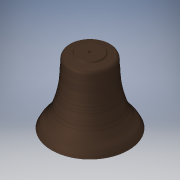
# Autodesk Inventor part: bell
Saved by Autodesk Inventor 2017 (Build 210142000, 142)
## iProperties
Created: 2016-09-29
Part Number: bell
Material: Bronze, Cast
Document SubType Name: Modeling
Designer: canti021
Density: 8.45 g/cm^3
Appearance: Bronze - Satin
Author: canti021
Autodesk Inventor part; units mm, degrees
ref_plane "YZ Plane" through (0, 0, 0) normal (1, 0, 0) x (0, 1, 0)
ref_plane "XZ Plane" through (0, 0, 0) normal (0, 1, 0) x (-1, 0, 0)
ref_plane "XY Plane" through (0, 0, 0) normal (0, 0, 1) x (1, 0, 0)
sketch "Sketch1" plane through (0, 0, 0) normal (0, 0, 1) x (1, 0, 0)
  spline S0 degree 3 poles (58.871, 16.2187) (58.8456, 16.6364) (59.2227, 17.7302) (62.2401, 23.533) (64.3081, 27.5098) (66, 31.0198) (66, 31.3331) (66, 31.6465) (68.4469, 36.5488) (71.4375, 42.2273) (76.7576, 52.3288) (77.7094, 54.0452) (83.4201, 63.8339) (84.9574, 66.469) (90.7691, 73.7771) (96.3349, 80.0741) (106.446, 91.5134) (114.75, 101.5516) (114.75, 102.335) (114.75, 102.5632) (115.2804, 103.3406) (115.9287, 104.0625) (117.7509, 106.0915) (128.1618, 122.2601) (129.8128, 125.625) (130.6224, 127.275) (132.2051, 130.0773) (133.3299, 131.8523) (137.2192, 137.9897) (150.75, 163.3632) (150.75, 164.5191) (150.75, 164.8886) (151.7405, 167.2573) (152.951, 169.783) (155.5846, 175.2773) (161.25, 190.7483) (161.25, 192.4455) (161.25, 193.1071) (161.7267, 194.7118) (162.3093, 196.0117) (162.8919, 197.3115) (164.1292, 201.4125) (165.0589, 205.125) (165.9886, 208.8375) (167.0014, 212.2125) (167.3095, 212.625) (167.6177, 213.0375) (168.591, 216.3598) (169.4725, 220.0078) (170.3539, 223.6558) (171.359, 227.1996) (171.706, 227.8828) (172.555, 229.5544) (174.7488, 237.242) (174.7546, 238.5659) (174.757, 239.1484) (175.2636, 240.592) (175.88, 241.7739) (176.4963, 242.9557) (177.6864, 246.837) (178.5246, 250.3989) (179.3627, 253.9607) (180.3404, 257.55) (180.6973, 258.375) (181.3815, 259.9569) (182.4138, 264.9065) (183.7475, 273) (184.1893, 275.6812) (184.8551, 278.55) (185.2271, 279.375) (185.599, 280.2) (186.6498, 285.0938) (187.5622, 290.25) (188.4745, 295.4062) (189.4794, 299.9625) (189.7952, 300.375) (190.111, 300.7875) (191.11, 306.3562) (192.0153, 312.75) (192.9205, 319.1438) (193.9326, 324.7125) (194.2645, 325.125) (194.5964, 325.5375) (195.244, 328.575) (195.7037, 331.875) (196.9806, 341.041) (198.6765, 352.8509) (199.8503, 360.75) (200.4326, 364.6688) (201.3057, 374.625) (201.7907, 382.875) (202.2756, 391.125) (202.9691, 398.4399) (203.3319, 399.1302) (203.6947, 399.8206) (204.6695, 416.9551) (205.4982, 437.2069) (206.327, 457.4587) (207.3134, 474.6126) (207.6904, 475.3267) (208.0675, 476.0408) (208.7597, 486.4125) (209.2287, 498.375) (210.504, 530.9028) (211.2343, 542.5727) (212.0952, 544.1776) (212.5221, 544.9737) (213.6114, 547.4813) (214.5157, 549.75) (216.8217, 555.5352) (221.1847, 561.067) (225.8758, 564.1535) (229.4678, 566.5169) (230.7149, 566.876) (238.125, 567.6802) (242.6625, 568.1727) (247.3875, 568.8781) (248.625, 569.2477) (249.8625, 569.6174) (257.2875, 570.6295) (265.125, 571.4968) (282.6702, 573.4384) (285.3766, 574.4859) (287.4793, 580.1489) (288.2336, 582.1805) (289.2088, 584.2742) (289.6466, 584.8016) (290.2812, 585.5662) (300.6399, 585.7215) (340.7837, 585.5677) (357.5641, 585.5035) (374.3446, 585.4392) (391.125, 585.375) (391.125, 581.7967) (391.125, 578.2456) (391.125, 574.6824) (391.125, 571.1192) (391.125, 567.5645) (391.125, 563.9878) (376.9718, 563.9894) (362.4025, 563.9788) (347.8331, 563.9682) (333.2637, 563.9576) (318.6944, 563.947) (304.125, 563.9364) (303.375, 562.426) (302.625, 560.9155) (301.875, 559.405) (300.6375, 556.9128) (299.2875, 554.5967) (298.875, 554.2583) (297.0424, 552.7548) (281.0236, 551.2893) (261, 550.7932) (253.875, 550.6167) (246.75, 550.4402) (239.625, 550.2637) (238.4663, 549.2882) (237.3075, 548.3127) (236.1488, 547.3372) (233.3231, 544.9584) (232.446, 543.6029) (231.4613, 540.0937) (230.7951, 537.7193) (230.25, 534.6797) (230.25, 533.339) (230.25, 531.9983) (229.9145, 530.2745) (229.5045, 529.5084) (229.0945, 528.7422) (228.21, 515.6863) (227.539, 500.4952) (226.868, 485.3041) (226.0173, 467.9812) (225.6487, 462) (225.28, 456.0188) (224.6956, 446.5688) (224.35, 441) (224.0044, 435.4312) (223.1662, 417.5438) (222.4875, 401.25) (221.8087, 384.9562) (220.9394, 370.4438) (220.5558, 369) (220.1721, 367.5562) (219.4736, 360.975) (219.0035, 354.375) (217.773, 337.0987) (216.3606, 322.3014) (215.8179, 321) (215.5598, 320.3812) (214.6315, 313.4625) (213.7549, 305.625) (212.8783, 297.7875) (211.8736, 290.7) (211.5221, 289.875) (210.8262, 288.2412) (209.4857, 280.6339) (208.1954, 270.9971) (207.7442, 267.6268) (207.1219, 264.6174) (206.8125, 264.3096) (206.5031, 264.0018) (206.25, 262.9976) (206.25, 262.078) (206.25, 259.787) (203.3245, 244.4781) (202.5325, 242.625) (201.713, 240.7073) (198.4367, 227.761) (196.0792, 217.125) (195.0735, 212.5875) (193.9209, 208.2) (193.5177, 207.375) (193.1146, 206.55) (192.0614, 203.021) (191.1772, 199.5329) (190.293, 196.0447) (189.3074, 192.6697) (188.9869, 192.0329) (188.6665, 191.396) (187.5573, 187.1625) (186.5221, 182.625) (184.5781, 174.1044) (181.7392, 163.8658) (177.8918, 151.5) (176.6726, 147.5812) (174.7608, 141.3375) (173.6434, 137.625) (172.526, 133.9125) (171.3569, 130.5375) (171.0454, 130.125) (170.7338, 129.7125) (169.8961, 127.5188) (169.1837, 125.25) (167.9712, 121.3882) (160.907, 104.0319) (157.126, 95.625) (156.1984, 93.5625) (155.0081, 90.525) (154.481, 88.875) (153.9538, 87.225) (153.1026, 85.2) (152.5894, 84.375) (152.0761, 83.55) (151.4054, 82.0312) (151.0988, 81) (150.7922, 79.9688) (148.9852, 76.3085) (147.0832, 72.8661) (145.1812, 69.4237) (141.6, 62.7675) (139.125, 58.0745) (136.65, 53.3815) (132.2821, 46.1097) (129.4185, 41.915) (124.941, 35.3561) (123.7334, 34.0892) (120.7935, 32.8663) (118.9133, 32.0843) (116.3625, 30.9613) (115.125, 30.3708) (113.8875, 29.7804) (110.85, 28.5885) (108.375, 27.7223) (105.9, 26.8562) (102.6348, 25.4882) (101.119, 24.6825) (97.8316, 22.9351) (89.7823, 20.718) (78, 18.3146) (68.7056, 16.4187) (64.2733, 15.411) (61.8226, 14.6364) (60.8676, 14.3345) (59.9258, 14.5607) (59.3753, 15.2241) (59.3753, 15.2241) (58.8964, 15.801) (58.871, 16.2187) knots 3 3 3 3 4 5 6 7 8 9 10 11 12 13 14 15 16 17 18 19 20 21 22 23 24 25 26 27 28 29 30 31 32 33 34 35 36 37 38 39 40 41 42 43 44 45 46 47 48 49 50 51 52 53 54 55 56 57 58 59 60 61 62 63 64 65 66 67 68 69 70 71 72 73 74 75 76 77 78 79 80 81 82 83 84 85 86 87 88 89 90 91 92 93 94 95 96 97 98 99 100 101 102 103 104 105 106 107 108 109 110 111 112 113 114 115 116 117 118 119 120 121 122 123 124 125 126 127 128 129 130 131 132 133 134 135 136 137 138 139 140 141 142 143 144 145 146 147 148 149 150 151 152 153 154 155 156 157 158 159 160 161 162 163 164 165 166 167 168 169 170 171 172 173 174 175 176 177 178 179 180 181 182 183 184 185 186 187 188 189 190 191 192 193 194 195 196 197 198 199 200 201 202 203 204 205 206 207 208 209 210 211 212 213 214 215 216 217 218 219 220 221 222 223 224 225 226 227 228 229 230 231 232 233 234 235 236 237 238 239 240 241 242 243 244 245 246 247 248 249 250 251 252 253 254 255 256 257 258 259 260 261 262 263 264 265 266 267 268 269 270 271 272 273 274 275 276 277 278 279 280 280 280 280
  line L0 (58.871, 16.2187) -> (58.8456, 16.6364) construction
  line L1 (58.8456, 16.6364) -> (59.2227, 17.7302) construction
  line L2 (59.2227, 17.7302) -> (62.2401, 23.533) construction
  line L3 (62.2401, 23.533) -> (64.3081, 27.5098) construction
  line L4 (64.3081, 27.5098) -> (66, 31.0198) construction
  line L5 (66, 31.0198) -> (66, 31.3331) construction
  line L6 (66, 31.3331) -> (66, 31.6465) construction
  line L7 (66, 31.6465) -> (68.4469, 36.5488) construction
  line L8 (68.4469, 36.5488) -> (71.4375, 42.2273) construction
  line L9 (71.4375, 42.2273) -> (76.7576, 52.3288) construction
  line L10 (76.7576, 52.3288) -> (77.7094, 54.0452) construction
  line L11 (77.7094, 54.0452) -> (83.4201, 63.8339) construction
  line L12 (83.4201, 63.8339) -> (84.9574, 66.469) construction
  line L13 (84.9574, 66.469) -> (90.7691, 73.7771) construction
  line L14 (90.7691, 73.7771) -> (96.3349, 80.0741) construction
  line L15 (96.3349, 80.0741) -> (106.446, 91.5134) construction
  line L16 (106.446, 91.5134) -> (114.75, 101.5516) construction
  line L17 (114.75, 101.5516) -> (114.75, 102.335) construction
  line L18 (114.75, 102.335) -> (114.75, 102.5632) construction
  line L19 (114.75, 102.5632) -> (115.2804, 103.3406) construction
  line L20 (115.2804, 103.3406) -> (115.9287, 104.0625) construction
  line L21 (115.9287, 104.0625) -> (117.7509, 106.0915) construction
  line L22 (117.7509, 106.0915) -> (128.1618, 122.2601) construction
  line L23 (128.1618, 122.2601) -> (129.8128, 125.625) construction
  line L24 (129.8128, 125.625) -> (130.6224, 127.275) construction
  line L25 (130.6224, 127.275) -> (132.2051, 130.0773) construction
  line L26 (132.2051, 130.0773) -> (133.3299, 131.8523) construction
  line L27 (133.3299, 131.8523) -> (137.2192, 137.9897) construction
  line L28 (137.2192, 137.9897) -> (150.75, 163.3632) construction
  line L29 (150.75, 163.3632) -> (150.75, 164.5191) construction
  line L30 (150.75, 164.5191) -> (150.75, 164.8886) construction
  line L31 (150.75, 164.8886) -> (151.7405, 167.2573) construction
  line L32 (151.7405, 167.2573) -> (152.951, 169.783) construction
  line L33 (152.951, 169.783) -> (155.5846, 175.2773) construction
  line L34 (155.5846, 175.2773) -> (161.25, 190.7483) construction
  line L35 (161.25, 190.7483) -> (161.25, 192.4455) construction
  line L36 (161.25, 192.4455) -> (161.25, 193.1071) construction
  line L37 (161.25, 193.1071) -> (161.7267, 194.7118) construction
  line L38 (161.7267, 194.7118) -> (162.3093, 196.0117) construction
  line L39 (162.3093, 196.0117) -> (162.8919, 197.3115) construction
  line L40 (162.8919, 197.3115) -> (164.1292, 201.4125) construction
  line L41 (164.1292, 201.4125) -> (165.0589, 205.125) construction
  line L42 (165.0589, 205.125) -> (165.9886, 208.8375) construction
  line L43 (165.9886, 208.8375) -> (167.0014, 212.2125) construction
  line L44 (167.0014, 212.2125) -> (167.3095, 212.625) construction
  line L45 (167.3095, 212.625) -> (167.6177, 213.0375) construction
  line L46 (167.6177, 213.0375) -> (168.591, 216.3598) construction
  line L47 (168.591, 216.3598) -> (169.4725, 220.0078) construction
  line L48 (169.4725, 220.0078) -> (170.3539, 223.6558) construction
  line L49 (170.3539, 223.6558) -> (171.359, 227.1996) construction
  line L50 (171.359, 227.1996) -> (171.706, 227.8828) construction
  line L51 (171.706, 227.8828) -> (172.555, 229.5544) construction
  line L52 (172.555, 229.5544) -> (174.7488, 237.242) construction
  line L53 (174.7488, 237.242) -> (174.7546, 238.5659) construction
  line L54 (174.7546, 238.5659) -> (174.757, 239.1484) construction
  line L55 (174.757, 239.1484) -> (175.2636, 240.592) construction
  line L56 (175.2636, 240.592) -> (175.88, 241.7739) construction
  line L57 (175.88, 241.7739) -> (176.4963, 242.9557) construction
  line L58 (176.4963, 242.9557) -> (177.6864, 246.837) construction
  line L59 (177.6864, 246.837) -> (178.5246, 250.3989) construction
  line L60 (178.5246, 250.3989) -> (179.3627, 253.9607) construction
  line L61 (179.3627, 253.9607) -> (180.3404, 257.55) construction
  line L62 (180.3404, 257.55) -> (180.6973, 258.375) construction
  line L63 (180.6973, 258.375) -> (181.3815, 259.9569) construction
  line L64 (181.3815, 259.9569) -> (182.4138, 264.9065) construction
  line L65 (182.4138, 264.9065) -> (183.7475, 273) construction
  line L66 (183.7475, 273) -> (184.1893, 275.6812) construction
  line L67 (184.1893, 275.6812) -> (184.8551, 278.55) construction
  line L68 (184.8551, 278.55) -> (185.2271, 279.375) construction
  line L69 (185.2271, 279.375) -> (185.599, 280.2) construction
  line L70 (185.599, 280.2) -> (186.6498, 285.0938) construction
  line L71 (186.6498, 285.0938) -> (187.5622, 290.25) construction
  line L72 (187.5622, 290.25) -> (188.4745, 295.4062) construction
  line L73 (188.4745, 295.4062) -> (189.4794, 299.9625) construction
  line L74 (189.4794, 299.9625) -> (189.7952, 300.375) construction
  line L75 (189.7952, 300.375) -> (190.111, 300.7875) construction
  line L76 (190.111, 300.7875) -> (191.11, 306.3562) construction
  line L77 (191.11, 306.3562) -> (192.0153, 312.75) construction
  line L78 (192.0153, 312.75) -> (192.9205, 319.1438) construction
  line L79 (192.9205, 319.1438) -> (193.9326, 324.7125) construction
  line L80 (193.9326, 324.7125) -> (194.2645, 325.125) construction
  line L81 (194.2645, 325.125) -> (194.5964, 325.5375) construction
  line L82 (194.5964, 325.5375) -> (195.244, 328.575) construction
  line L83 (195.244, 328.575) -> (195.7037, 331.875) construction
  line L84 (195.7037, 331.875) -> (196.9806, 341.041) construction
  line L85 (196.9806, 341.041) -> (198.6765, 352.8509) construction
  line L86 (198.6765, 352.8509) -> (199.8503, 360.75) construction
  line L87 (199.8503, 360.75) -> (200.4326, 364.6688) construction
  line L88 (200.4326, 364.6688) -> (201.3057, 374.625) construction
  line L89 (201.3057, 374.625) -> (201.7907, 382.875) construction
  line L90 (201.7907, 382.875) -> (202.2756, 391.125) construction
  line L91 (202.2756, 391.125) -> (202.9691, 398.4399) construction
  line L92 (202.9691, 398.4399) -> (203.3319, 399.1302) construction
  line L93 (203.3319, 399.1302) -> (203.6947, 399.8206) construction
  line L94 (203.6947, 399.8206) -> (204.6695, 416.9551) construction
  line L95 (204.6695, 416.9551) -> (205.4982, 437.2069) construction
  line L96 (205.4982, 437.2069) -> (206.327, 457.4587) construction
  line L97 (206.327, 457.4587) -> (207.3134, 474.6126) construction
  line L98 (207.3134, 474.6126) -> (207.6904, 475.3267) construction
  line L99 (207.6904, 475.3267) -> (208.0675, 476.0408) construction
  line L100 (208.0675, 476.0408) -> (208.7597, 486.4125) construction
  line L101 (208.7597, 486.4125) -> (209.2287, 498.375) construction
  line L102 (209.2287, 498.375) -> (210.504, 530.9028) construction
  line L103 (210.504, 530.9028) -> (211.2343, 542.5727) construction
  line L104 (211.2343, 542.5727) -> (212.0952, 544.1776) construction
  line L105 (212.0952, 544.1776) -> (212.5221, 544.9737) construction
  line L106 (212.5221, 544.9737) -> (213.6114, 547.4813) construction
  line L107 (213.6114, 547.4813) -> (214.5157, 549.75) construction
  line L108 (214.5157, 549.75) -> (216.8217, 555.5352) construction
  line L109 (216.8217, 555.5352) -> (221.1847, 561.067) construction
  line L110 (221.1847, 561.067) -> (225.8758, 564.1535) construction
  line L111 (225.8758, 564.1535) -> (229.4678, 566.5169) construction
  line L112 (229.4678, 566.5169) -> (230.7149, 566.876) construction
  line L113 (230.7149, 566.876) -> (238.125, 567.6802) construction
  line L114 (238.125, 567.6802) -> (242.6625, 568.1727) construction
  line L115 (242.6625, 568.1727) -> (247.3875, 568.8781) construction
  line L116 (247.3875, 568.8781) -> (248.625, 569.2477) construction
  line L117 (248.625, 569.2477) -> (249.8625, 569.6174) construction
  line L118 (249.8625, 569.6174) -> (257.2875, 570.6295) construction
  line L119 (257.2875, 570.6295) -> (265.125, 571.4968) construction
  line L120 (265.125, 571.4968) -> (282.6702, 573.4384) construction
  line L121 (282.6702, 573.4384) -> (285.3766, 574.4859) construction
  line L122 (285.3766, 574.4859) -> (287.4793, 580.1489) construction
  line L123 (287.4793, 580.1489) -> (288.2336, 582.1805) construction
  line L124 (288.2336, 582.1805) -> (289.2088, 584.2742) construction
  line L125 (289.2088, 584.2742) -> (289.6466, 584.8016) construction
  line L126 (289.6466, 584.8016) -> (290.2812, 585.5662) construction
  line L127 (290.2812, 585.5662) -> (300.6399, 585.7215) construction
  line L128 (300.6399, 585.7215) -> (340.7837, 585.5677) construction
  line L129 (340.7837, 585.5677) -> (357.5641, 585.5035) construction
  line L130 (357.5641, 585.5035) -> (374.3446, 585.4392) construction
  line L131 (374.3446, 585.4392) -> (391.125, 585.375) construction
  line L132 (391.125, 585.375) -> (391.125, 581.7967) construction
  line L133 (391.125, 581.7967) -> (391.125, 578.2456) construction
  line L134 (391.125, 578.2456) -> (391.125, 574.6824) construction
  line L135 (391.125, 574.6824) -> (391.125, 571.1192) construction
  line L136 (391.125, 571.1192) -> (391.125, 567.5645) construction
  line L137 (391.125, 567.5645) -> (391.125, 563.9878) construction
  line L138 (391.125, 563.9878) -> (376.9718, 563.9894) construction
  line L139 (376.9718, 563.9894) -> (362.4025, 563.9788) construction
  line L140 (362.4025, 563.9788) -> (347.8331, 563.9682) construction
  line L141 (347.8331, 563.9682) -> (333.2637, 563.9576) construction
  line L142 (333.2637, 563.9576) -> (318.6944, 563.947) construction
  line L143 (318.6944, 563.947) -> (304.125, 563.9364) construction
  line L144 (304.125, 563.9364) -> (303.375, 562.426) construction
  line L145 (303.375, 562.426) -> (302.625, 560.9155) construction
  line L146 (302.625, 560.9155) -> (301.875, 559.405) construction
  line L147 (301.875, 559.405) -> (300.6375, 556.9128) construction
  line L148 (300.6375, 556.9128) -> (299.2875, 554.5967) construction
  line L149 (299.2875, 554.5967) -> (298.875, 554.2583) construction
  line L150 (298.875, 554.2583) -> (297.0424, 552.7548) construction
  line L151 (297.0424, 552.7548) -> (281.0236, 551.2893) construction
  line L152 (281.0236, 551.2893) -> (261, 550.7932) construction
  line L153 (261, 550.7932) -> (253.875, 550.6167) construction
  line L154 (253.875, 550.6167) -> (246.75, 550.4402) construction
  line L155 (246.75, 550.4402) -> (239.625, 550.2637) construction
  line L156 (239.625, 550.2637) -> (238.4663, 549.2882) construction
  line L157 (238.4663, 549.2882) -> (237.3075, 548.3127) construction
  line L158 (237.3075, 548.3127) -> (236.1488, 547.3372) construction
  line L159 (236.1488, 547.3372) -> (233.3231, 544.9584) construction
  line L160 (233.3231, 544.9584) -> (232.446, 543.6029) construction
  line L161 (232.446, 543.6029) -> (231.4613, 540.0937) construction
  line L162 (231.4613, 540.0937) -> (230.7951, 537.7193) construction
  line L163 (230.7951, 537.7193) -> (230.25, 534.6797) construction
  line L164 (230.25, 534.6797) -> (230.25, 533.339) construction
  line L165 (230.25, 533.339) -> (230.25, 531.9983) construction
  line L166 (230.25, 531.9983) -> (229.9145, 530.2745) construction
  line L167 (229.9145, 530.2745) -> (229.5045, 529.5084) construction
  line L168 (229.5045, 529.5084) -> (229.0945, 528.7422) construction
  line L169 (229.0945, 528.7422) -> (228.21, 515.6863) construction
  line L170 (228.21, 515.6863) -> (227.539, 500.4952) construction
  line L171 (227.539, 500.4952) -> (226.868, 485.3041) construction
  line L172 (226.868, 485.3041) -> (226.0173, 467.9812) construction
  line L173 (226.0173, 467.9812) -> (225.6487, 462) construction
  line L174 (225.6487, 462) -> (225.28, 456.0188) construction
  line L175 (225.28, 456.0188) -> (224.6956, 446.5688) construction
  line L176 (224.6956, 446.5688) -> (224.35, 441) construction
  line L177 (224.35, 441) -> (224.0044, 435.4312) construction
  line L178 (224.0044, 435.4312) -> (223.1662, 417.5438) construction
  line L179 (223.1662, 417.5438) -> (222.4875, 401.25) construction
  line L180 (222.4875, 401.25) -> (221.8087, 384.9562) construction
  line L181 (221.8087, 384.9562) -> (220.9394, 370.4438) construction
  line L182 (220.9394, 370.4438) -> (220.5558, 369) construction
  line L183 (220.5558, 369) -> (220.1721, 367.5562) construction
  line L184 (220.1721, 367.5562) -> (219.4736, 360.975) construction
  line L185 (219.4736, 360.975) -> (219.0035, 354.375) construction
  line L186 (219.0035, 354.375) -> (217.773, 337.0987) construction
  line L187 (217.773, 337.0987) -> (216.3606, 322.3014) construction
  line L188 (216.3606, 322.3014) -> (215.8179, 321) construction
  line L189 (215.8179, 321) -> (215.5598, 320.3812) construction
  line L190 (215.5598, 320.3812) -> (214.6315, 313.4625) construction
  line L191 (214.6315, 313.4625) -> (213.7549, 305.625) construction
  line L192 (213.7549, 305.625) -> (212.8783, 297.7875) construction
  line L193 (212.8783, 297.7875) -> (211.8736, 290.7) construction
  line L194 (211.8736, 290.7) -> (211.5221, 289.875) construction
  line L195 (211.5221, 289.875) -> (210.8262, 288.2412) construction
  line L196 (210.8262, 288.2412) -> (209.4857, 280.6339) construction
  line L197 (209.4857, 280.6339) -> (208.1954, 270.9971) construction
  line L198 (208.1954, 270.9971) -> (207.7442, 267.6268) construction
  line L199 (207.7442, 267.6268) -> (207.1219, 264.6174) construction
  line L200 (207.1219, 264.6174) -> (206.8125, 264.3096) construction
  line L201 (206.8125, 264.3096) -> (206.5031, 264.0018) construction
  line L202 (206.5031, 264.0018) -> (206.25, 262.9976) construction
  line L203 (206.25, 262.9976) -> (206.25, 262.078) construction
  line L204 (206.25, 262.078) -> (206.25, 259.787) construction
  line L205 (206.25, 259.787) -> (203.3245, 244.4781) construction
  line L206 (203.3245, 244.4781) -> (202.5325, 242.625) construction
  line L207 (202.5325, 242.625) -> (201.713, 240.7073) construction
  line L208 (201.713, 240.7073) -> (198.4367, 227.761) construction
  line L209 (198.4367, 227.761) -> (196.0792, 217.125) construction
  line L210 (196.0792, 217.125) -> (195.0735, 212.5875) construction
  line L211 (195.0735, 212.5875) -> (193.9209, 208.2) construction
  line L212 (193.9209, 208.2) -> (193.5177, 207.375) construction
  line L213 (193.5177, 207.375) -> (193.1146, 206.55) construction
  line L214 (193.1146, 206.55) -> (192.0614, 203.021) construction
  line L215 (192.0614, 203.021) -> (191.1772, 199.5329) construction
  line L216 (191.1772, 199.5329) -> (190.293, 196.0447) construction
  line L217 (190.293, 196.0447) -> (189.3074, 192.6697) construction
  line L218 (189.3074, 192.6697) -> (188.9869, 192.0329) construction
  line L219 (188.9869, 192.0329) -> (188.6665, 191.396) construction
  line L220 (188.6665, 191.396) -> (187.5573, 187.1625) construction
  line L221 (187.5573, 187.1625) -> (186.5221, 182.625) construction
  line L222 (186.5221, 182.625) -> (184.5781, 174.1044) construction
  line L223 (184.5781, 174.1044) -> (181.7392, 163.8658) construction
  line L224 (181.7392, 163.8658) -> (177.8918, 151.5) construction
  line L225 (177.8918, 151.5) -> (176.6726, 147.5812) construction
  line L226 (176.6726, 147.5812) -> (174.7608, 141.3375) construction
  line L227 (174.7608, 141.3375) -> (173.6434, 137.625) construction
  line L228 (173.6434, 137.625) -> (172.526, 133.9125) construction
  line L229 (172.526, 133.9125) -> (171.3569, 130.5375) construction
  line L230 (171.3569, 130.5375) -> (171.0454, 130.125) construction
  line L231 (171.0454, 130.125) -> (170.7338, 129.7125) construction
  line L232 (170.7338, 129.7125) -> (169.8961, 127.5188) construction
  line L233 (169.8961, 127.5188) -> (169.1837, 125.25) construction
  line L234 (169.1837, 125.25) -> (167.9712, 121.3882) construction
  line L235 (167.9712, 121.3882) -> (160.907, 104.0319) construction
  line L236 (160.907, 104.0319) -> (157.126, 95.625) construction
  line L237 (157.126, 95.625) -> (156.1984, 93.5625) construction
  line L238 (156.1984, 93.5625) -> (155.0081, 90.525) construction
  line L239 (155.0081, 90.525) -> (154.481, 88.875) construction
  line L240 (154.481, 88.875) -> (153.9538, 87.225) construction
  line L241 (153.9538, 87.225) -> (153.1026, 85.2) construction
  line L242 (153.1026, 85.2) -> (152.5894, 84.375) construction
  line L243 (152.5894, 84.375) -> (152.0761, 83.55) construction
  line L244 (152.0761, 83.55) -> (151.4054, 82.0312) construction
  line L245 (151.4054, 82.0312) -> (151.0988, 81) construction
  line L246 (151.0988, 81) -> (150.7922, 79.9688) construction
  line L247 (150.7922, 79.9688) -> (148.9852, 76.3085) construction
  line L248 (148.9852, 76.3085) -> (147.0832, 72.8661) construction
  line L249 (147.0832, 72.8661) -> (145.1812, 69.4237) construction
  line L250 (145.1812, 69.4237) -> (141.6, 62.7675) construction
  line L251 (141.6, 62.7675) -> (139.125, 58.0745) construction
  line L252 (139.125, 58.0745) -> (136.65, 53.3815) construction
  line L253 (136.65, 53.3815) -> (132.2821, 46.1097) construction
  line L254 (132.2821, 46.1097) -> (129.4185, 41.915) construction
  line L255 (129.4185, 41.915) -> (124.941, 35.3561) construction
  line L256 (124.941, 35.3561) -> (123.7334, 34.0892) construction
  line L257 (123.7334, 34.0892) -> (120.7935, 32.8663) construction
  line L258 (120.7935, 32.8663) -> (118.9133, 32.0843) construction
  line L259 (118.9133, 32.0843) -> (116.3625, 30.9613) construction
  line L260 (116.3625, 30.9613) -> (115.125, 30.3708) construction
  line L261 (115.125, 30.3708) -> (113.8875, 29.7804) construction
  line L262 (113.8875, 29.7804) -> (110.85, 28.5885) construction
  line L263 (110.85, 28.5885) -> (108.375, 27.7223) construction
  line L264 (108.375, 27.7223) -> (105.9, 26.8562) construction
  line L265 (105.9, 26.8562) -> (102.6348, 25.4882) construction
  line L266 (102.6348, 25.4882) -> (101.119, 24.6825) construction
  line L267 (101.119, 24.6825) -> (97.8316, 22.9351) construction
  line L268 (97.8316, 22.9351) -> (89.7823, 20.718) construction
  line L269 (89.7823, 20.718) -> (78, 18.3146) construction
  line L270 (78, 18.3146) -> (68.7056, 16.4187) construction
  line L271 (68.7056, 16.4187) -> (64.2733, 15.411) construction
  line L272 (64.2733, 15.411) -> (61.8226, 14.6364) construction
  line L273 (61.8226, 14.6364) -> (60.8676, 14.3345) construction
  line L274 (60.8676, 14.3345) -> (59.9258, 14.5607) construction
  line L275 (59.9258, 14.5607) -> (59.3753, 15.2241) construction
  line L276 (59.3753, 15.2241) -> (59.3753, 15.2241) construction
  line L277 (59.3753, 15.2241) -> (58.8964, 15.801) construction
  line L278 (58.8964, 15.801) -> (58.871, 16.2187) construction
  line L279 (391.125, 578.2456) -> (391.2196, 578.2456)
  line L280 (391.2196, 578.2456) -> (391.2196, 567.9264)
  line L281 (391.2196, 567.9264) -> (391.125, 567.9264)
  line L282 (391.125, 567.9264) -> (391.125, 578.2456)
  point P0 (0, 0)
  constraints: 8 end point, 6 vertical, 2 parallel, 2 vertical alignment, 1 coincident, 1 horizontal, 1 perpendicular, 1 other
revolve "Revolution1" add sketch "Sketch1" angle 360 about axis through (391.2196, 578.2456, 0) along (0, -1, 0) contours S0
sketch "Sketch4" plane through (0, 0, 0) normal (0, 1, 0) x (-1, 0, 0)
  circle A0 centre (-391.2196, 0) radius 12.7448
  circle A1 centre (-391.2196, 0) radius 332.3486 projected
  point P0 (0, 0)
  point P1 (-58.871, 0)
  constraints: 1 centre point, 1 horizontal alignment, 1 other
hole "Hole1" at (391.2196, 0, 0) direction (0, 1, 0) diameter 25 end through all
body "Solid1"
